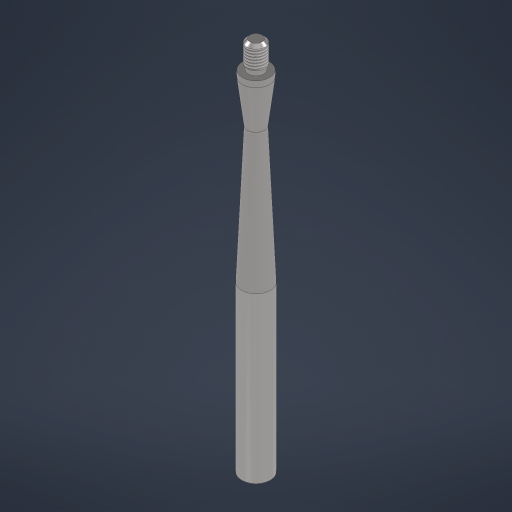
# Autodesk Inventor part: HM1-001
Saved by Autodesk Inventor 2024.3 (Build 283343000, 343)
## iProperties
Created: 2023-12-03
Part Number: HM1-001
Material: Steel, Alloy
Document SubType Name: Modeling
Designer: fablabadmin
Density: 7.73 g/cm^3
Appearance: Semi-Polished
Description: Shaft
Author: fablabadmin
Autodesk Inventor part; units mm, degrees
ref_plane "YZ Plane" through (0, 0, 0) normal (1, 0, 0) x (0, 1, 0)
ref_plane "XZ Plane" through (0, 0, 0) normal (0, 1, 0) x (-1, 0, 0)
ref_plane "XY Plane" through (0, 0, 0) normal (0, 0, 1) x (1, 0, 0)
sketch "Sketch1" plane through (0, 0, 0) normal (0, 0, 1) x (1, 0, 0)
  line L0 (0, 0) -> (-9.5, 0)
  line L1 (-9.5, 0) -> (-9.5, 110)
  line L2 (-9.5, 110) -> (-5.5705, 200)
  line L3 (-5.5705, 200) -> (-9, 228)
  line L4 (-9, 228) -> (-9, 232)
  line L5 (-9, 232) -> (-5, 232)
  line L6 (-5, 232) -> (-5, 235)
  line L7 (-5, 235) -> (-6, 235.5774)
  line L8 (-6, 235.5774) -> (-6, 250)
  line L9 (-6, 250) -> (0, 250)
  line L10 (0, 250) -> (0, 0)
  line L11 (0, -50) -> (0, 300) projected
  line L12 (-11.4, 0) -> (1.9, 0) projected
  dimension "d0" = 250
  dimension "d1" = 19
  dimension "d2" = 110
  dimension "d5" = 11.141
  dimension "d6" = 12
  dimension "d7" = 3
  dimension "d9" = 18
  dimension "d10" = 4
  dimension "d11" = 10
  dimension "d12" = 60
  dimension "d13" = 18
  dimension "d14" = 2.5
  dimension "d16" = 6.983
  dimension "d17" = 200
  dimension "d18" = 232
  dimension "d19" = 50
  dimension "d20" = 14.4227
  constraints: 22 end point, 4 perpendicular, 2 parallel, 1 horizontal, 1 vertical
  measures "d0" distance of L9.end L0.start
  measures "d1" diameter of L1 L11
  measures "d2" distance of L0.end L1.end
  measures "d5" diameter of L2.end L11
  measures "d6" diameter of L8 L11
  measures "d7" distance of L5.end L6.end
  measures "d9" distance between parallel lines of L5 L9
  measures "d10" distance of L3.end L4.end
  measures "d11" diameter of L6 L11
  measures "d12" angle of L6 L7
  measures "d13" diameter of L4 L11
  measures "d14" angle of L10 L2
  measures "d16" angle of L11 L3
  measures "d17" vertical distance of L2.end L0.end
  measures "d18" vertical distance of L0.end L4.end
  measures "d19" vertical distance of L2.end L8.end
  measures "d20" distance of L7.end L8.end
revolve "Revolution1" add sketch "Sketch1" angle 360 about axis through (0, -10, 0) along (0, 1, 0)
thread "Thread1" size "M12x1.75" class "6g" standard "ISO Metric profile" full length
sketch "Sketch2" plane through (0, 0, 0) normal (0, -1, 0) x (1, 0, 0)
  circle A0 centre (0, 0) radius 9.5 projected
  constraints: 1 coincident
hole "Hole1" at (0, 0, 0) direction (0, 1, 0) diameter 15 depth 80 tip angle 118 countersink diameter 15.5 countersink angle 90
chamfer "Chamfer2" distance 2 angle 45 1 edges at (6, 250, 0)
chamfer "Chamfer3" distance 1 angle 45 1 edges at (9.5, 0, 0)
body "Solid1"
